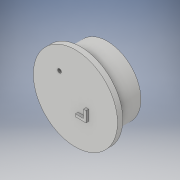
# Autodesk Inventor part: ChipMount
Saved by Autodesk Inventor 2019 (Build 230136000, 136)
## iProperties
Created: 2019-05-13
Part Number: ChipMount
Material: Generic
Document SubType Name: Modeling
Designer: aorfi
Density: 1 g/cm^3
Appearance: Default
Author: aorfi
Autodesk Inventor part; units mm, degrees
ref_plane "YZ Plane" through (0, 0, 0) normal (1, 0, 0) x (0, 1, 0)
ref_plane "XZ Plane" through (0, 0, 0) normal (0, 1, 0) x (-1, 0, 0)
ref_plane "XY Plane" through (0, 0, 0) normal (0, 0, 1) x (1, 0, 0)
sketch "Sketch1" plane through (0, 0, 0) normal (0, 0, 1) x (1, 0, 0)
  line L0 (-20, -20) -> (20, -20)
  line L1 (20, -20) -> (20, 20)
  line L2 (20, 20) -> (-20, 20)
  line L3 (-20, 20) -> (-20, -20)
  line L4 (-20, -20) -> (20, 20) construction
  line L5 (20, -20) -> (-20, 20) construction
  circle A0 centre (0, 0) radius 15.875
  dimension "d0" = 40
  dimension "d51" = 31.75
  constraints: 12 end point, 2 midpoint, 2 parallel, 2 perpendicular, 1 centre point, 1 coincident, 1 horizontal
  measures "d0" distance of L1.end L2.end
  measures "d51" diameter of A0
extrude "Extrusion1" add sketch "Sketch1" along normal blind 2 contours A0
sketch "Sketch4" plane through (0, 0, 2) normal (0, 0, 1) x (1, 0, 0)
  line L0 (-4, 4) -> (4, 4)
  line L1 (4, 4) -> (4, -4)
  line L2 (4, -4) -> (-4, -4)
  line L3 (-4, -4) -> (-4, 4)
  line L4 (-4, 4) -> (4, -4) construction
  line L5 (4, 4) -> (-4, -4) construction
  line L6 (4, -1) -> (5, -1)
  line L7 (5, -1) -> (5, -5)
  line L8 (5, -5) -> (1, -5)
  line L9 (1, -5) -> (1, -4)
  point P0 (0, 0)
  point P1 (0, 0)
  point P2 (0, 0)
  point P3 (-6, 6)
  point P4 (0, 0)
  dimension "d16" = 8
  dimension "d17" = 1
  dimension "d18" = 4
  dimension "d30" = 6
  dimension "d31" = 6
  constraints: 20 end point, 7 perpendicular, 4 midpoint, 2 coincident, 2 horizontal, 2 parallel, 2 point on line
  measures "d16" distance of L1.end L2.end
  measures "d17" distance of L6.start L6.end
  measures "d18" distance of L6.end L7.end
  measures "d30" horizontal distance of point (0, 0) point (-6, 6)
  measures "d31" horizontal distance of point (0, 0) point (-6, 6)
sketch "Sketch9" plane through (0, 0, 0) normal (0, 0, -1) x (-1, 0, 0)
  circle A0 centre (0, 0) radius 12.7
  dimension "d52" = 25.4
  constraints: 1 centre point, 1 coincident
  measures "d52" diameter of A0
extrude "Extrusion6" add sketch "Sketch9" along normal blind 10
extrude "Extrusion7" add sketch "Sketch4" along normal blind 1 contours L6 L7 L8 L9 L2 L1
hole "Hole4" at (-6, 6, 2) direction (0, 0, -1) diameter 1.425 depth 5.692 tip angle 118 thread size "1-64 UNC" class "2B" standard "ANSI Unified Screw Threads"
equation "\"d31\" = d30"
body "Solid1"
